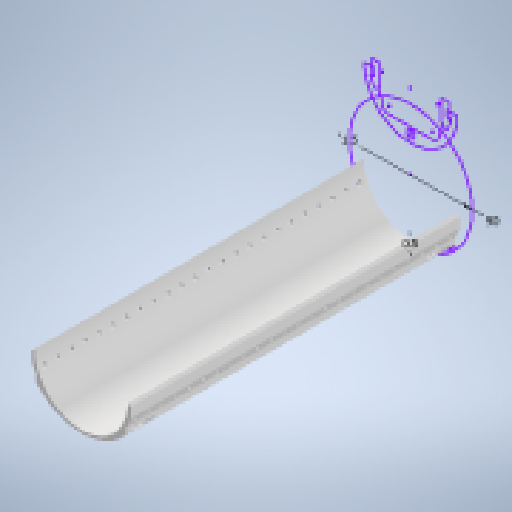
# Autodesk Inventor part: Base
Saved by Autodesk Inventor 2023 (Build 270158030, 158C)
## iProperties
Created: 2023-03-20
Part Number: Base
Material: Generic
Document SubType Name: Modeling
Designer: sqa4002
Density: 1 g/cm^3
Appearance: Default
Author: sqa4002
Autodesk Inventor part; units mm, degrees
ref_plane "YZ Plane" through (0, 0, 0) normal (1, 0, 0) x (0, 1, 0)
ref_plane "XZ Plane" through (0, 0, 0) normal (0, 1, 0) x (-1, 0, 0)
ref_plane "XY Plane" through (0, 0, 0) normal (0, 0, 1) x (1, 0, 0)
sketch "Sketch1" plane through (0, 0, 0) normal (0, 0, 1) x (1, 0, 0)
  circle A0 centre (0, 0) radius 45
  arc A1 (-35, -28.2843) -> (35, -28.2843) centre (0, 0) ccw
  arc A2 (-33.0492, -28.2843) -> (33.0492, -28.2843) centre (0, 0) ccw
  arc A3 (-32.3883, -28.2843) -> (32.3883, -28.2843) centre (0, 0) ccw
  point P0 (0, -45)
  dimension "d0" = 90
  dimension "d2" = 1.5
  dimension "d3" = 0.5
  constraints: 10 point on circle, 4 centre point, 1 coincident
  measures "d0" diameter of A0
  measures "d2" radial gap between concentric circles of A0 A2
  measures "d3" radial gap between concentric circles of A2 A3
sketch "Sketch2" plane through (0, 0, 0) normal (0, 0, 1) x (1, 0, 0)
  line L0 (-16.1473, 30.376) -> (15.8527, 30.376)
  arc A0 (-21.1473, 35.376) -> (-16.1473, 30.376) centre (-16.1473, 35.376) ccw
  line L1 (-21.1473, 35.376) -> (-21.1473, 37.376)
  line L2 (-21.1473, 37.376) -> (-23.7395, 42.8844)
  line L3 (-23.7395, 42.8844) -> (-26.6351, 41.5218)
  line L4 (-26.6351, 41.5218) -> (-29.786, 48.2174)
  line L5 (-29.786, 48.2174) -> (-26.6599, 49.6885)
  arc A1 (-26.6599, 49.6885) -> (-26.5827, 49.5903) centre (-20.3312, 54.5821) ccw
  line L6 (-26.5827, 49.5903) -> (-26.3285, 49.7224)
  line L7 (-26.3285, 49.7224) -> (-26.3285, 54.3755)
  line L8 (-26.3285, 54.3755) -> (-34.1473, 54.3755)
  arc A2 (-34.1473, 54.3755) -> (-0.1473, 20.3755) centre (-0.1473, 54.3755) ccw
  arc A3 (-0.1473, 20.3755) -> (33.8527, 54.3755) centre (-0.1473, 54.3755) ccw
  line L9 (26.034, 54.3755) -> (33.8527, 54.3755)
  line L10 (26.034, 50.0041) -> (26.034, 54.3755)
  line L11 (26.4435, 49.7913) -> (26.034, 50.0041)
  arc A4 (26.3654, 49.6885) -> (26.4435, 49.7913) centre (20.0366, 54.5821) ccw
  line L12 (29.4912, 48.2175) -> (26.3654, 49.6885)
  line L13 (26.3405, 41.5223) -> (29.4912, 48.2175)
  line L14 (23.4451, 42.8848) -> (26.3405, 41.5223)
  line L15 (20.8527, 37.376) -> (23.4451, 42.8848)
  line L16 (20.8527, 35.376) -> (20.8527, 37.376)
  arc A5 (15.8527, 30.376) -> (20.8527, 35.376) centre (15.8527, 35.376) ccw
  arc A6 (29.699, 48.4374) -> (29.7027, 48.4388) centre (29.3527, 49.3755) ccw
  line L17 (29.7027, 48.4388) -> (29.7027, 48.4355)
  line L18 (29.699, 48.4374) -> (29.7027, 48.4355)
  arc A7 (-0.1473, 22.876) -> (-0.1473, 28.876) centre (-0.1473, 25.876) ccw
  arc A8 (-0.1473, 28.876) -> (-0.1473, 22.876) centre (-0.1473, 25.876) ccw
  line L19 (-28.4414, 49.7865) -> (-28.4414, 59.9755)
  line L20 (-28.4414, 59.9755) -> (-22.4414, 59.9755)
  line L21 (-22.4414, 44.3755) -> (-22.4414, 59.9755)
  line L22 (-22.4414, 44.3755) -> (-23.5898, 42.5659)
  line L23 (23.2952, 42.5659) -> (22.1468, 44.3755)
  line L24 (22.1468, 44.3755) -> (22.1468, 59.9755)
  line L25 (28.1468, 59.9755) -> (22.1468, 59.9755)
  line L26 (28.1468, 49.3755) -> (28.1468, 59.9755)
  point P0 (0, 0)
  point P1 (-0.1473, 54.3755)
  dimension "d8" = 50.402
  dimension "d6" = 0
  dimension "d7" = 44.5882
  dimension "d9" = 4.5
  dimension "d10" = 4.5
  dimension "d11" = 32
  dimension "d12" = -25.876
  dimension "d13" = 52.3625
  dimension "d14" = 68
  dimension "d15" = 180
  dimension "d16" = -30.376
  dimension "d17" = 22.4414
  dimension "d18" = 34.1473
  constraints: 50 end point, 18 point on circle, 9 centre point, 6 other
  measures "d6" distance of A3.centre A2.centre
  measures "d7" distance between parallel lines of L24 L21
  measures "d9" distance from line of L0 A8.centre
  measures "d10" distance from line of L0 A7.centre
  measures "d11" distance of A5.centre A0.centre
  measures "d12" vertical distance of point (0, 0) A8.centre
  measures "d13" distance between parallel lines of L10 L7
  measures "d14" distance of L9.end L8.end
  measures "d15" angle of L9 L8
  measures "d16" distance from line of point (0, 0) L0
  measures "d17" distance from line of point (0, 0) L21
  measures "d18" horizontal distance of point (0, 0) L8.end
sketch "Sketch3" plane through (0, 0, 0) normal (0, 0, 1) x (1, 0, 0)
  arc A0 (-34, -7) -> (34, -7) centre (0, -7) ccw
  line L0 (-34, -7) -> (-26.1812, -7)
  line L1 (34, -7) -> (26.1812, -7)
  line L2 (-26.1812, -7) -> (-26.1812, -11.6531)
  line L3 (26.1812, -7) -> (26.1812, -11.6531)
  line L4 (-26.1812, -11.6531) -> (-29.5916, -13.258)
  line L5 (26.1812, -11.6531) -> (29.5916, -13.258)
  line L6 (-29.5916, -13.258) -> (-26.4408, -19.9537)
  line L7 (29.5916, -13.258) -> (26.4408, -19.9537)
  line L8 (-26.4408, -19.9537) -> (-23.5453, -18.5911)
  line L9 (26.4408, -19.9537) -> (23.5453, -18.5911)
  line L10 (-23.5453, -18.5911) -> (-20.6171, -24.8136)
  line L11 (23.5453, -18.5911) -> (20.6171, -24.8136)
  line L12 (-20.6171, -24.8136) -> (-20.6171, -26.8136)
  line L13 (20.6171, -24.8136) -> (20.6171, -26.8136)
  arc A1 (-20.6171, -26.8136) -> (-15.6171, -31.8136) centre (-15.6171, -26.8136) ccw
  arc A2 (15.6171, -31.8136) -> (20.6171, -26.8136) centre (15.6171, -26.8136) ccw
  line L14 (-15.6171, -31.8136) -> (15.6171, -31.8136)
  line L15 (-34, -7) -> (-31.5, -7) construction
  line L16 (-35.7678, -8.7678) -> (-35.7678, -16.1644)
  arc A3 (-32.3883, -28.2843) -> (32.3883, -28.2843) centre (0, 0) ccw projected
  line L17 (-35.7678, -16.1644) -> (-32.75, -22.9227)
  line L18 (-32.75, -22.9227) -> (-32.75, -27.8646)
  line L19 (-32.75, -27.8646) -> (-32.3883, -28.2843)
  line L20 (35.7678, -8.7678) -> (35.7678, -16.1644)
  line L21 (35.7678, -16.1644) -> (32.75, -22.9227)
  line L22 (32.75, -22.9227) -> (32.75, -27.8646)
  line L23 (32.75, -27.8646) -> (32.3883, -28.2843)
  line L24 (34, -7) -> (35.7678, -7)
  line L25 (35.7678, -7) -> (35.7678, -8.7678)
  line L26 (-35.7678, -8.7678) -> (-35.7678, -7)
  line L27 (-35.7678, -7) -> (-34, -7)
  dimension "d19" = 68
  dimension "d20" = 34
  dimension "d21" = 7.8188
  dimension "d22" = 7.8188
  dimension "d23" = 4.6531
  dimension "d24" = 4.6531
  dimension "d25" = 3.7692
  dimension "d26" = 3.7692
  dimension "d27" = 115.201
  dimension "d28" = 115.201
  dimension "d29" = 7.4
  dimension "d30" = 90
  dimension "d31" = 90
  dimension "d32" = 3.2
  dimension "d33" = 90
  dimension "d34" = 3.2
  dimension "d35" = 90
  dimension "d36" = 6.877
  dimension "d37" = 90
  dimension "d38" = 6.877
  dimension "d39" = 90
  dimension "d40" = 2
  dimension "d43" = 5
  dimension "d49" = 5
  dimension "d50" = 31.2343
  dimension "d51" = 31.8136
  dimension "d52" = 2.5
  dimension "d54" = 2.5
  constraints: 56 end point, 7 vertical, 6 point on circle, 5 horizontal, 3 centre point, 2 parallel, 1 collinear, 1 perpendicular
  measures "d19" distance of L0.start L1.start
  measures "d20" radius of A0
  measures "d21" distance of L0.start L0.end
  measures "d22" distance of L1.start L1.end
  measures "d23" distance of L0.end L2.end
  measures "d24" distance of L1.end L3.end
  measures "d25" distance of L2.end L4.end
  measures "d26" distance of L3.end L5.end
  measures "d27" angle of L4 L2
  measures "d28" angle of L5 L3
  measures "d29" distance of L4.end L6.end
  measures "d30" angle of L6 L4
  measures "d31" angle of L7 L5
  measures "d32" distance of L6.end L8.end
  measures "d33" angle of L8 L6
  measures "d34" distance of L7.end L9.end
  measures "d35" angle of L7 L9
  measures "d36" distance of L8.end L10.end
  measures "d37" angle of L10 L8
  measures "d38" distance of L9.end L11.end
  measures "d39" angle of L11 L9
  measures "d40" distance of L10.end L12.end
  measures "d43" radius of A1
  measures "d49" radius of A2
  measures "d50" distance of L14.start L14.end
  measures "d51" distance from line of L14 point (0, 0)
  measures "d52" distance of L0.start L16.start
  measures "d54" distance of L1.start L20.start
extrude "Extrusion1" add sketch "Sketch3" along normal blind 240 contours A0 L24 L25 L20 L21 L22 L23 A3 L19 L18 L17 L16 L26 L27
sketch "Sketch5" plane through (35.7678, -16.1644, 240) normal (0.9131044, -0.4077258, 0) x (0, 0, -1)
  line L0 (240, -7.4015) -> (240, 0) projected
  line L1 (240, 0) -> (0, 0) projected
  line L2 (0, -7.4015) -> (0, 0) projected
  line L3 (240, -7.4015) -> (0, -7.4015) projected
  circle A0 centre (235, -3.7007) radius 1.5
  circle A1 centre (225, -3.7007) radius 1.5
  circle A2 centre (215, -3.7007) radius 1.5
  circle A3 centre (205, -3.7007) radius 1.5
  circle A4 centre (195, -3.7007) radius 1.5
  circle A5 centre (185, -3.7007) radius 1.5
  circle A6 centre (175, -3.7007) radius 1.5
  circle A7 centre (165, -3.7007) radius 1.5
  circle A8 centre (155, -3.7007) radius 1.5
  circle A9 centre (145, -3.7007) radius 1.5
  circle A10 centre (135, -3.7007) radius 1.5
  circle A11 centre (125, -3.7007) radius 1.5
  circle A12 centre (115, -3.7007) radius 1.5
  circle A13 centre (105, -3.7007) radius 1.5
  circle A14 centre (95, -3.7007) radius 1.5
  circle A15 centre (85, -3.7007) radius 1.5
  circle A16 centre (75, -3.7007) radius 1.5
  circle A17 centre (65, -3.7007) radius 1.5
  circle A18 centre (55, -3.7007) radius 1.5
  circle A19 centre (45, -3.7007) radius 1.5
  circle A20 centre (35, -3.7007) radius 1.5
  circle A21 centre (25, -3.7007) radius 1.5
  circle A22 centre (15, -3.7007) radius 1.5
  circle A23 centre (5, -3.7007) radius 1.5
  point P0 (240, 0.1763)
  dimension "d66" = 3
  dimension "d67" = 5
  dimension "d70" = 10
  constraints: 24 centre point, 1 horizontal, 46 other
  measures "d66" diameter of A0
  measures "d67" distance from line of L0 A0.centre
  measures "d70" distance of A0.centre A1.centre
sketch "Sketch6" plane through (-32.75, -22.9227, 0) normal (-0.9131044, -0.4077258, 0) x (0, 0, 1)
  line L0 (0, 7.4015) -> (0, 0) projected
  line L1 (0, 0) -> (240, 0) projected
  line L2 (240, 7.4015) -> (240, 0) projected
  line L3 (0, 7.4015) -> (240, 7.4015) projected
  circle A0 centre (5, 3.7007) radius 1.5
  circle A1 centre (15, 3.7007) radius 1.5
  circle A2 centre (25, 3.7007) radius 1.5
  circle A3 centre (35, 3.7007) radius 1.5
  circle A4 centre (45, 3.7007) radius 1.5
  circle A5 centre (55, 3.7007) radius 1.5
  circle A6 centre (65, 3.7007) radius 1.5
  circle A7 centre (75, 3.7007) radius 1.5
  circle A8 centre (85, 3.7007) radius 1.5
  circle A9 centre (95, 3.7007) radius 1.5
  circle A10 centre (105, 3.7007) radius 1.5
  circle A11 centre (115, 3.7007) radius 1.5
  circle A12 centre (125, 3.7007) radius 1.5
  circle A13 centre (135, 3.7007) radius 1.5
  circle A14 centre (145, 3.7007) radius 1.5
  circle A15 centre (155, 3.7007) radius 1.5
  circle A16 centre (165, 3.7007) radius 1.5
  circle A17 centre (175, 3.7007) radius 1.5
  circle A18 centre (185, 3.7007) radius 1.5
  circle A19 centre (195, 3.7007) radius 1.5
  circle A20 centre (205, 3.7007) radius 1.5
  circle A21 centre (215, 3.7007) radius 1.5
  circle A22 centre (225, 3.7007) radius 1.5
  circle A23 centre (235, 3.7007) radius 1.5
  point P0 (0, 7.5778)
  dimension "d75" = 3
  dimension "d76" = 5
  dimension "d79" = 10
  constraints: 24 centre point, 1 horizontal, 46 other
  measures "d75" diameter of A0
  measures "d76" distance from line of L0 A0.centre
  measures "d79" distance of A0.centre A1.centre
extrude "Extrusion2" cut sketch "Sketch6" against normal up to surface contours A0 | A1 | A2 | A3 | A4 | A5 | A6 | A7 | A8 | A9 | A10 | A11 | A12 | A13 | A14 | A15 | A16 | A17 | A18 | A19 | A20 | A21 | A22 | A23 round surface about axis through (0, -7, 0) along (0, 0, 1) radius 34 far side no
extrude "Extrusion3" cut sketch "Sketch5" against normal up to surface contours A0 | A1 | A2 | A3 | A4 | A5 | A6 | A7 | A8 | A9 | A10 | A11 | A12 | A13 | A14 | A15 | A16 | A17 | A18 | A19 | A20 | A21 | A22 | A23 round surface about axis through (0, -7, 0) along (0, 0, 1) radius 34 far side no
sketch "Sketch7" plane through (-32.75, -27.8646, 0) normal (-1, 0, 0) x (0, 0, 1)
  line L0 (0, 0) -> (240, 0) projected
  line L1 (0, 4.9419) -> (0, 0) projected
  line L2 (5, 1.5) -> (20, 1.5) construction
  line L3 (5, 1) -> (20, 1)
  line L4 (20, 2) -> (5, 2)
  arc A0 (5, 2) -> (5, 1) centre (5, 1.5) ccw
  arc A1 (20, 1) -> (20, 2) centre (20, 1.5) ccw
  line L5 (0, -15.1354) -> (0, -0.4196) projected
  line L6 (0, -15.1354) -> (0, -0.4196) projected
  line L7 (0, -15.6354) -> (0, -0.4196) projected
  line L8 (0, 0) -> (0, 4.9419) projected
  point P0 (0, 27.8646)
  point P1 (12.5, 1.5)
  point P2 (0, -0.4196)
  dimension "d88" = 15
  dimension "d89" = 1
  dimension "d90" = 1
  dimension "d91" = 5
  constraints: 8 end point, 4 point on circle, 4 tangent, 2 centre point, 2 parallel, 1 midpoint
  measures "d88" distance of L2.start L2.end
  measures "d89" diameter of A1
  measures "d90" distance between parallel lines of L0 L3
  measures "d91" distance from line of L1 L2.start
sketch "Sketch8" plane through (0, 0, 0) normal (0, 0, -1) x (-1, 0, 0)
  line L0 (-32.75, -27.8646) -> (-32.75, -22.9227) projected
  line L1 (32.75, -22.9227) -> (32.75, -27.8646) projected
  line L2 (32.75, -26.8646) -> (32.75, -25.8646) projected
  arc A0 (-32.75, -26.3646) -> (32.75, -26.3646) centre (0, -0.0694) ccw
  point P0 (0, 0)
  dimension "d92" = 42
  constraints: 2 point on circle, 1 centre point, 1 point on line
  measures "d92" radius of A0
sweep "Sweep1" cut profiles "Sketch7" path "Sketch8" keep normal constant yes path curves A0
sketch "Sketch9" plane through (-32.75, -27.8646, 0) normal (-1, 0, 0) x (0, 0, 1)
  line L0 (235, 1.5) -> (220, 1.5) construction
  line L1 (235, 2) -> (220, 2)
  line L2 (220, 1) -> (235, 1)
  arc A0 (235, 1) -> (235, 2) centre (235, 1.5) ccw
  arc A1 (220, 2) -> (220, 1) centre (220, 1.5) ccw
  line L3 (235, 1.5) -> (250, 1.5) construction
  line L4 (240, 4.9419) -> (240, 0) projected
  line L5 (0, 0) -> (240, 0) projected
  point P0 (0, 27.8646)
  point P1 (227.5, 1.5)
  point P2 (240, 2.471)
  dimension "d95" = 15
  dimension "d96" = 180
  dimension "d97" = 1
  dimension "d98" = 5
  dimension "d99" = 1
  constraints: 10 end point, 4 point on circle, 4 tangent, 2 centre point, 2 horizontal, 2 midpoint, 1 collinear, 1 parallel
  measures "d95" distance of L0.start L0.end
  measures "d96" angle of L0 L3
  measures "d97" diameter of A1
  measures "d98" horizontal distance of point (240, 2.471) L0.start
  measures "d99" distance between parallel lines of L5 L2
sketch "Sketch10" plane through (0, 0, 240) normal (0, 0, 1) x (1, 0, 0)
  line L0 (32.75, -27.8646) -> (32.75, -22.9227) projected
  line L1 (-32.75, -22.9227) -> (-32.75, -27.8646) projected
  line L2 (-32.75, -25.8646) -> (-32.75, -26.8646) projected
  arc A0 (-32.75, -26.3646) -> (32.75, -26.3646) centre (0, -0.0694) ccw
  point P0 (0, 0)
  dimension "d100" = 42
  constraints: 2 point on circle, 1 centre point, 1 point on line
  measures "d100" radius of A0
sweep "Sweep2" cut profiles "Sketch9" path "Sketch10" keep normal constant yes path curves A0
sketch "Sketch11" plane through (0, 0, 0) normal (0, 0, -1) x (-1, 0, 0)
  arc A0 (-34, -7) -> (34, -7) centre (0, -7) ccw projected
  line L0 (-34, -7) -> (-34, 1)
  line L1 (34, -7) -> (35.7678, -8.7678) projected
  line L2 (34, -7) -> (34, 1)
  line L3 (34, 1) -> (-34, 1)
  line L4 (-34, 1) -> (-34, 27)
  line L5 (34, 1) -> (34, 27)
  arc A1 (-34, 27) -> (34, 27) centre (0, 27) ccw
  point P0 (0, 0)
  dimension "d103" = 8
  dimension "d104" = 26
  dimension "d105" = 26
  dimension "d106" = 34
  constraints: 10 end point, 4 vertical, 2 point on circle, 1 centre point, 1 horizontal, 1 tangent
  measures "d103" distance of L0.start L0.end
  measures "d104" distance of L0.end L4.end
  measures "d105" distance of L2.end L5.end
  measures "d106" radius of A1
body "Solid1"
